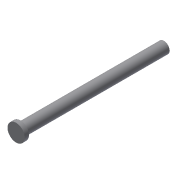
# Autodesk Inventor part: 4mmScrew
Saved by Autodesk Inventor 2014 (Build 180170000, 170)
## iProperties
Created: 2015-01-20
Part Number: 4mmScrew
Material: Generic
Document SubType Name: Modeling
Designer: Peele
Density: 1 g/cm^3
Appearance: Default
Author: Peele
Autodesk Inventor part; units mm, degrees
ref_plane "YZ Plane" through (0, 0, 0) normal (1, 0, 0) x (0, 1, 0)
ref_plane "XZ Plane" through (0, 0, 0) normal (0, 1, 0) x (-1, 0, 0)
ref_plane "XY Plane" through (0, 0, 0) normal (0, 0, 1) x (1, 0, 0)
sketch "Sketch1" plane through (0, 0, 0) normal (0, 0, 1) x (1, 0, 0)
  line L0 (0, 0) -> (-3, 0)
  line L1 (-3, 0) -> (-3, 1.5)
  line L2 (-3, 1.5) -> (-2, 1.5)
  line L3 (-2, 1.5) -> (-2, 51.5)
  line L4 (-2, 51.5) -> (0, 51.5)
  line L5 (0, 51.5) -> (0, 0)
  dimension "d0" = 2
  dimension "d1" = 3
  dimension "d2" = 1.5
  dimension "d3" = 50
  constraints: 12 end point, 3 parallel, 2 perpendicular, 1 horizontal
  measures "d0" distance between parallel lines of L3 L5
  measures "d1" distance of L0.start L0.end
  measures "d2" distance of L0.end L1.end
  measures "d3" distance of L2.end L3.end
revolve "Revolution1" add sketch "Sketch1" angle 360 about axis through (0, 51.5, 0) along (0, -1, 0)
body "Solid1"
